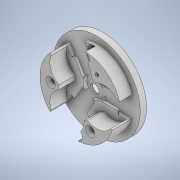
# Autodesk Inventor part: akkuhalterung_deckel_2
Saved by Autodesk Inventor 2022 (Build 260153000, 153)
## iProperties
Created: 2021-04-19
Part Number: akkuhalterung_deckel_2
Material: Generisch
Document SubType Name: Modeling
Designer: g.schardt
Density: 1 g/cm^3
Appearance: Vorgabe
Author: g.schardt
Autodesk Inventor part; units mm, degrees
ref_plane "YZ Plane" through (0, 0, 0) normal (1, 0, 0) x (0, 1, 0)
ref_plane "XZ Plane" through (0, 0, 0) normal (0, 1, 0) x (-1, 0, 0)
ref_plane "XY Plane" through (0, 0, 0) normal (0, 0, 1) x (1, 0, 0)
sketch "Skizze1" plane through (0, 0, 0) normal (0, 0, 1) x (1, 0, 0)
  circle A0 centre (0, 0) radius 20.4
  dimension "d0" = 40.8
  constraints: 1 centre point, 1 coincident
  measures "d0" diameter of A0
extrude "Extrusion1" add sketch "Skizze1" along normal blind 8
sketch "Skizze2" plane through (0, 0, 8) normal (0, 0, 1) x (1, 0, 0)
  circle A0 centre (10.95, 0) radius 9.45
  circle A1 centre (0, 0) radius 20.4 projected
  circle A2 centre (-5.475, 9.483) radius 9.45
  circle A3 centre (-5.475, -9.483) radius 9.45
  point P0 (1.5, 0)
  point P1 (-0.75, 1.299)
  point P2 (-0.75, -1.299)
  dimension "d3" = 18.9
  dimension "d6" = 360
  constraints: 3 horizontal alignment, 19 other
extrude "Extrusion2" cut sketch "Skizze2" against normal blind 4.5 contours A0 | A2 | A3
sketch "Skizze3" plane through (-5.475, 9.483, 8) normal (0, 0, 1) x (1, 0, 0)
  circle A0 centre (5.475, -9.483) radius 10
  dimension "d10" = 20
  constraints: 1 centre point, 1 coincident
  measures "d10" diameter of A0
extrude "Extrusion3" cut sketch "Skizze3" against normal blind 4.5
sketch "Skizze4" plane through (0, 0, 3.5) normal (0, 0, 1) x (1, 0, 0)
  line L0 (4.95, 5.75) -> (24.95, 5.75)
  line L1 (24.95, 5.75) -> (24.95, -5.75)
  line L2 (24.95, -5.75) -> (4.95, -5.75)
  line L3 (4.95, -5.75) -> (4.95, 5.75)
  circle A0 centre (0, 0) radius 20.4 projected
  arc A1 (5.9635, -8.0273) -> (5.9635, 8.0273) centre (10.95, 0) ccw projected
  arc A2 (5.9635, 8.0273) -> (3.9701, 9.1782) centre (0, 0) ccw projected
  arc A3 (20.4, 0) -> (5.9635, 8.0273) centre (10.95, 0) ccw projected
  arc A4 (20.4, 0) -> (-10.2, 17.6669) centre (0, 0) ccw projected
  arc A5 (3.9701, 9.1782) -> (-10.2, 17.6669) centre (-5.475, 9.483) ccw projected
  arc A6 (3.9701, -9.1782) -> (5.9635, -8.0273) centre (0, 0) ccw projected
  arc A7 (-10.2, -17.6669) -> (3.9701, -9.1782) centre (-5.475, -9.483) ccw projected
  arc A8 (-9.9336, 1.1509) -> (-9.9336, -1.1509) centre (0, 0) ccw projected
  arc A9 (-10.2, -17.6669) -> (20.4, 0) centre (0, 0) ccw projected
  arc A10 (5.9635, -8.0273) -> (20.4, 0) centre (10.95, 0) ccw projected
  arc A11 (-10.2, 17.6669) -> (-9.9336, 1.1509) centre (-5.475, 9.483) ccw projected
  arc A12 (-10.2, 17.6669) -> (-10.2, -17.6669) centre (0, 0) ccw projected
  arc A13 (-9.9336, -1.1509) -> (-10.2, -17.6669) centre (-5.475, -9.483) ccw projected
  point P0 (24.95, 0)
  point P1 (19.5729, 5.75)
  point P2 (18.4493, 5.75)
  point P3 (19.5729, -5.75)
  point P4 (18.4493, -5.75)
  dimension "d13" = 20
  dimension "d14" = 11.5
  dimension "d33" = 6
  constraints: 8 end point, 2 parallel, 1 horizontal, 1 horizontal alignment, 1 midpoint, 1 perpendicular, 1 other
  measures "d13" distance of L1.end L2.end
  measures "d14" distance of L0.end L1.end
  measures "d33" distance from line of L3 A1.centre
extrude "Extrusion4" cut sketch "Skizze4" against normal blind 2 contours L0 A1 L2 L3 | L0 A0 A1 | L0 L1 L2 A0 | A0 L2 A1
sketch "Skizze25" plane through (0, 0, 8) normal (0, 0, 1) x (1, 0, 0)
  arc A0 (19.5729, -5.75) -> (19.5729, 5.75) centre (0, 0) ccw projected
  line L0 (4.95, 5.75) -> (19.5729, 5.75) projected
  line L1 (4.95, -5.75) -> (4.95, 5.75) projected
  line L2 (19.5729, -5.75) -> (4.95, -5.75) projected
extrude "Extrusion21" cut sketch "Skizze25" against normal blind 4.5
sketch "Skizze6" plane through (0, 0, 3.5) normal (0, 0, 1) x (1, 0, 0)
  line L0 (4.95, 5.75) -> (13.95, 5.75)
  line L1 (13.95, 3.95) -> (4.95, 3.95)
  line L2 (4.95, 3.95) -> (4.95, 5.75)
  line L3 (18.4493, -5.75) -> (4.95, -5.75) projected
  line L4 (4.95, -5.75) -> (13.95, -5.75)
  line L5 (13.95, -3.95) -> (4.95, -3.95)
  line L6 (4.95, -3.95) -> (4.95, -5.75)
  line L7 (13.95, 3.95) -> (13.95, 5.75)
  line L8 (13.95, -3.95) -> (13.95, -5.75)
  point P0 (0, 0)
  point P1 (19.5729, 5.75)
  point P2 (8.1815, -5.75)
  point P3 (8.1815, -5.75)
  dimension "d240" = 1.8
  dimension "d241" = 1.8
  dimension "d242" = 9
  dimension "d243" = 9
  constraints: 16 end point, 2 horizontal, 2 parallel, 1 perpendicular, 1 point on line
  measures "d240" distance of L1.end L0.start
  measures "d241" distance of L5.end L3.end
  measures "d242" distance of L1.start L1.end
  measures "d243" distance of L5.start L5.end
extrude "Extrusion6" add sketch "Skizze6" against normal blind 1.3
pattern_circular "Runde Anordnung1" count 3 over 360 about axis through (0, 0, 0) along (0, 0, 1) of "Extrusion4", "Extrusion6", "Extrusion21"
sketch "Skizze7" plane through (0, 0, 3.5) normal (0, 0, 1) x (1, 0, 0)
  circle A0 centre (0, 0) radius 5.5
  dimension "d40" = 11
  constraints: 1 centre point, 1 coincident
  measures "d40" diameter of A0
extrude "Extrusion7" cut sketch "Skizze7" against normal blind 2
sketch "Skizze26" plane through (0, 0, 8) normal (0, 0, 1) x (1, 0, 0)
  line L0 (-4.8068, 19.8256) -> (-4.245, 18.8526) projected
  arc A0 (3.9701, 9.1782) -> (-4.245, 18.8526) centre (-5.475, 9.483) ccw projected
  arc A1 (5.9635, 8.0273) -> (3.9701, 9.1782) centre (0, 0) ccw projected
  arc A2 (18.4493, 5.75) -> (5.9635, 8.0273) centre (10.95, 0) ccw projected
  line L1 (18.4493, 5.75) -> (19.5729, 5.75) projected
  arc A3 (19.5729, 5.75) -> (-4.8068, 19.8256) centre (0, 0) ccw projected
  line L2 (-4.245, -18.8526) -> (-4.8068, -19.8256) projected
  arc A4 (-4.8068, -19.8256) -> (19.5729, -5.75) centre (0, 0) ccw projected
  line L3 (19.5729, -5.75) -> (18.4493, -5.75) projected
  arc A5 (5.9635, -8.0273) -> (18.4493, -5.75) centre (10.95, 0) ccw projected
  arc A6 (3.9701, -9.1782) -> (5.9635, -8.0273) centre (0, 0) ccw projected
  arc A7 (-4.245, -18.8526) -> (3.9701, -9.1782) centre (-5.475, -9.483) ccw projected
  line L4 (-14.7661, -14.0756) -> (-14.2043, -13.1026) projected
  arc A8 (-9.9336, -1.1509) -> (-14.2043, -13.1026) centre (-5.475, -9.483) ccw projected
  arc A9 (-9.9336, 1.1509) -> (-9.9336, -1.1509) centre (0, 0) ccw projected
  arc A10 (-14.2043, 13.1026) -> (-9.9336, 1.1509) centre (-5.475, 9.483) ccw projected
  line L5 (-14.2043, 13.1026) -> (-14.7661, 14.0756) projected
  arc A11 (-14.7661, 14.0756) -> (-14.7661, -14.0756) centre (0, 0) ccw projected
extrude "Extrusion22" add sketch "Skizze26" along normal blind 0.5
sketch "Skizze33" plane through (0, 0, 0) normal (0, 0, -1) x (-1, 0, 0)
  circle A0 centre (0, 0) radius 20.4 projected
  circle A1 centre (0, 0) radius 24
  dimension "d165" = 48
  constraints: 1 centre point, 1 coincident
  measures "d165" diameter of A1
extrude "Extrusion25" add sketch "Skizze33" against normal blind 1.5
sketch "Skizze34" plane through (0, 0, 0) normal (0, 0, -1) x (-1, 0, 0)
  circle A0 centre (0, 0) radius 24 projected
  circle A1 centre (0, 0) radius 23
  dimension "d168" = 1
  constraints: 1 centre point
  measures "d168" radial gap between concentric circles of A0 A1
extrude "Extrusion26" add sketch "Skizze34" along normal blind 2
sketch "Skizze36" plane through (0, 0, 8.5) normal (0, 0, 1) x (1, 0, 0)
  line L0 (0, 0) -> (12, 20.7846) construction
  circle A0 centre (0, 0) radius 24 construction
  line L1 (0, 0) -> (24, 0) construction
  circle A1 centre (-14.5, 0) radius 1.75 construction
  circle A2 centre (0, 0) radius 14.5 construction
  point P0 (7.25, 12.5574)
  dimension "d181" = 60
  constraints: 4 end point, 2 point on circle, 1 centre point, 1 coincident, 1 equal length, 1 horizontal, 1 point on line, 2 other
  measures "d181" angle of L1 L0
hole "Bohrung8" at (7.25, 12.5574, 8.5) direction (0, 0, -1) diameter 1.8 end through all
sketch "Skizze38" plane through (0, 0, 8.5) normal (0, 0, 1) x (1, 0, 0)
  circle A0 centre (0, 0) radius 17.5
  point P0 (0, -17.5)
  point P1 (0, 17.5)
  dimension "d190" = 35
  constraints: 2 point on circle, 1 centre point, 1 coincident
  measures "d190" diameter of A0
hole "Bohrung9" at (0, -17.5, 8.5) at (0, 17.5, 8.5) direction (0, 0, -1) diameter 6 depth 5
sketch "Skizze40" plane through (0, 0, 3.5) normal (0, 0, 1) x (1, 0, 0)
  circle A0 centre (0, 0) radius 18 construction
  point P0 (0, 18)
  point P1 (0, -18)
  dimension "d200" = 36
  constraints: 2 point on circle, 1 centre point, 1 coincident
  measures "d200" diameter of A0
hole "Bohrung10" at (0, 18, 3.5) at (0, -18, 3.5) direction (0, 0, -1) diameter 3.2 depth 60 countersink diameter 5.2 countersink angle 90
sketch "Skizze41" plane through (0, 0, 8.5) normal (0, 0, 1) x (1, 0, 0)
  arc A0 (-2.8104, -18.5495) -> (-0.8291, -20.3831) centre (0, -17.5) ccw projected
  arc A1 (-4.245, -18.8526) -> (-2.8104, -18.5495) centre (-5.475, -9.483) ccw projected
  line L0 (-4.245, -18.8526) -> (-4.8068, -19.8256) projected
  arc A2 (-4.8068, -19.8256) -> (-0.8291, -20.3831) centre (0, 0) ccw projected
  arc A3 (-0.8291, 20.3831) -> (-2.8104, 18.5495) centre (0, 17.5) ccw projected
  arc A4 (-0.8291, 20.3831) -> (-4.8068, 19.8256) centre (0, 0) ccw projected
  line L1 (-4.8068, 19.8256) -> (-4.245, 18.8526) projected
  arc A5 (-2.8104, 18.5495) -> (-4.245, 18.8526) centre (-5.475, 9.483) ccw projected
extrude "Extrusion28" cut sketch "Skizze41" against normal up to surface (5 mm away)
sketch "Skizze42" plane through (0, 0, 1.5) normal (0, 0, 1) x (1, 0, 0)
  line L0 (0, 0) -> (-5, -8.6603) construction
  line L1 (0, 0) -> (10, 0) construction
  line L2 (-0.3988, -5.4855) -> (0.9458, -6.2618) projected
  point P0 (-1.225, -2.1218)
  dimension "d210" = 10
  dimension "d211" = 120
  dimension "d212" = 2.5
  constraints: 4 end point, 1 equal length, 1 horizontal, 1 point on line
  measures "d210" distance of L0.start L0.end
  measures "d211" angle of L0 L1
  measures "d212" distance from line of point (-1.225, -2.122) L2
hole "Bohrung11" at (-1.225, -2.1218, 1.5) direction (0, 0, -1) diameter 5 depth 80
sketch "Skizze45" plane through (0, 0, 8.5) normal (0, 0, 1) x (1, 0, 0)
  arc A0 (0.8291, -20.3831) -> (2.0003, -15.2642) centre (0, -17.5) ccw projected
  arc A1 (0.8291, -20.3831) -> (19.5729, -5.75) centre (0, 0) ccw projected
  line L0 (19.5729, -5.75) -> (18.4493, -5.75) projected
  arc A2 (5.9635, -8.0273) -> (18.4493, -5.75) centre (10.95, 0) ccw projected
  arc A3 (3.9701, -9.1782) -> (5.9635, -8.0273) centre (0, 0) ccw projected
  arc A4 (2.0003, -15.2642) -> (3.9701, -9.1782) centre (-5.475, -9.483) ccw projected
  arc A5 (-14.7661, 14.0756) -> (-14.7661, -14.0756) centre (0, 0) ccw projected
  line L1 (-14.7661, -14.0756) -> (-14.2043, -13.1026) projected
  arc A6 (-9.9336, -1.1509) -> (-14.2043, -13.1026) centre (-5.475, -9.483) ccw projected
  arc A7 (-9.9336, 1.1509) -> (-9.9336, -1.1509) centre (0, 0) ccw projected
  arc A8 (-14.2043, 13.1026) -> (-9.9336, 1.1509) centre (-5.475, 9.483) ccw projected
  line L2 (-14.2043, 13.1026) -> (-14.7661, 14.0756) projected
extrude "Extrusion29" add sketch "Skizze45" along normal blind 4
sketch "Skizze46" plane through (0, 0, 12.5) normal (0, 0, 1) x (1, 0, 0)
  point P0 (0, 0)
  point P1 (-14.5, 0)
  dimension "d226" = 14.5
  constraints: 1 horizontal alignment
  measures "d226" distance of point (0, 0) point (-14.5, 0)
hole "Bohrung12" at (-14.5, 0, 12.5) direction (0, 0, -1) diameter 2.3 end through all
chamfer "Fase1" distance 1.5 angle 45 1 edges at (-14.5, 1.15, 12.5)
pattern_circular "Runde Anordnung7" count 2 over 120 about axis through (0, 0, 0) along (0, 0, 1) of "Bohrung12", "Fase1"
chamfer "Fase2" distance 1 angle 45 6 edges at (13.95, 4.85, 2.2) (13.95, -4.85, 2.2) (-11.1752, -9.6561, 2.2) (-2.7748, -14.5061, 2.2) (-2.7748, 14.5061, 2.2) (-11.1752, 9.6561, 2.2)
sketch "Skizze47" plane through (0, 0, 0) normal (0, 0, -1) x (-1, 0, 0)
  circle A0 centre (0, 18) radius 1.6 projected
  circle A1 centre (0, -18) radius 1.6 projected
  circle A2 centre (0, 18) radius 1.6 projected
  circle A3 centre (0, 18) radius 3.25
  circle A4 centre (0, -18) radius 3.25
  point P0 (0, 0)
  dimension "d247" = 6.5
  dimension "d248" = 6.5
  constraints: 2 centre point, 2 coincident
  measures "d247" diameter of A3
  measures "d248" diameter of A4
extrude "Extrusion30" add sketch "Skizze47" along normal blind 0.5
